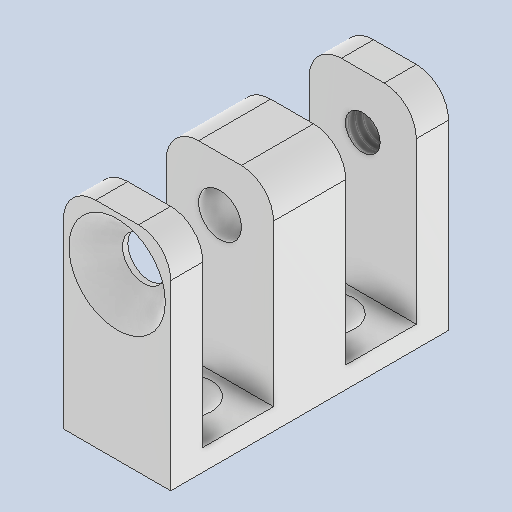
# Autodesk Inventor part: HalterUmlenkrolleDPL
Saved by Autodesk Inventor 2025 (Build 290162010, 162A)
## iProperties
Created: 2024-11-18
Part Number: HalterUmlenkrolleDPL
Material: PC/ABS-Kunststoff, 3DDruck, PLA
Document SubType Name: Modeling
Designer: Admin
Density: 1.1 g/cm^3
Appearance: Glatt - Weiß(2)
Mass: 2.7775 g
Surface Area: 22.2803 cm^2
Volume: 2.525 cm^3
Author: Admin
Autodesk Inventor part; units mm, degrees
ref_plane "YZ Plane" through (0, 0, 0) normal (1, 0, 0) x (0, 1, 0)
ref_plane "XZ Plane" through (0, 0, 0) normal (0, 1, 0) x (-1, 0, 0)
ref_plane "XY Plane" through (0, 0, 0) normal (0, 0, 1) x (1, 0, 0)
sketch "Skizze1" plane through (0, 0, 0) normal (0, 0, 1) x (1, 0, 0)
  line L0 (12.8939, 32.0057) -> (2.8939, 32.0057)
  line L1 (2.8939, 32.0057) -> (2.8939, 29.0057)
  line L2 (2.8939, 29.0057) -> (12.8939, 29.0057)
  line L3 (12.8939, 29.0057) -> (12.8939, 32.0057)
  line L4 (12.8939, 9.0723) -> (2.8939, 9.0723)
  line L5 (2.8939, 9.0723) -> (2.8939, 6.0723)
  line L6 (2.8939, 6.0723) -> (12.8939, 6.0723)
  line L7 (12.8939, 6.0723) -> (12.8939, 9.0723)
  line L8 (2.8939, 15.6723) -> (12.8939, 15.6723)
  line L9 (12.8939, 15.6723) -> (12.8939, 22.4057)
  line L10 (12.8939, 22.4057) -> (2.8939, 22.4057)
  line L11 (2.8939, 22.4057) -> (2.8939, 15.6723)
  line L12 (2.8939, 9.0723) -> (2.8939, 15.6723) construction
  line L13 (2.8939, 22.4057) -> (2.8939, 29.0057) construction
  point P0 (0, 0)
  point P1 (7.8939, 9.0723)
  dimension "d0" = 10
  dimension "d1" = 3
  dimension "d2" = 3
  dimension "d35" = 25.9333
  dimension "d38" = 6.6
  dimension "d39" = 6.7333
  constraints: 28 end point, 7 equal length, 4 collinear, 4 horizontal, 3 perpendicular, 2 vertical, 1 midpoint
  measures "d0" distance of L2.end L1.end
  measures "d1" distance of L0.end L1.end
  measures "d2" distance of L4.end L5.end
  measures "d35" distance between parallel lines of L0 L6
  measures "d38" distance of L8.start L4.end
  measures "d39" distance of L8.end L9.end
extrude "Extrusion1" add sketch "Skizze1" along normal blind 20
fillet "Rundung1" radius 3 6 edges at (12.8939, 7.5723, 20) (12.8939, 30.5057, 20) (2.8939, 30.5057, 20) (2.8939, 7.5723, 20) (12.8939, 19.039, 20) (2.8939, 19.039, 20)
sketch "Skizze2" plane through (2.8939, 6.0723, 0) normal (0, -1, 0) x (1, 0, 0)
  circle A0 centre (5, 15) radius 5 construction
  line L0 (10, 0) -> (10, 17) construction
  line L1 (0, 0) -> (0, 17) construction
  line L2 (3, 20) -> (7, 20) construction
  point P0 (-2.8939, 0)
  constraints: 3 tangent, 1 centre point
hole "Bohrung1" at (7.8939, 6.0723, 15) direction (0, 1, 0) diameter 3.242 end through all countersink diameter 9 countersink angle 90 thread size "M4x0.7" class "6H" standard "ISO Metric profile"
sketch "Skizze3" plane through (2.8939, 29.0057, 0) normal (0, -1, 0) x (1, 0, 0)
  line L0 (0, 0) -> (10, 0) projected
  line L1 (10, 0) -> (10, 2)
  line L2 (10, 0) -> (10, 17) projected
  line L3 (10, 2) -> (0, 2)
  line L4 (0, 0) -> (0, 17) projected
  point P0 (-2.8939, 0)
  dimension "d15" = 2
  constraints: 4 end point, 2 point on line, 1 perpendicular
  measures "d15" distance of L0.end L1.end
extrude "Extrusion2" add sketch "Skizze3" along normal through all
sketch "Skizze4" plane through (2.8939, 29.0057, 2) normal (0, 0, 1) x (1, 0, 0)
  line L0 (5, -16.6333) -> (10, -16.6333) construction
  line L1 (10, -16.6333) -> (10, 0) construction
  line L2 (10, -16.6333) -> (10, -19.9333) construction
  line L3 (5, -3.3) -> (0, -3.3) construction
  line L4 (0, 0) -> (0, -3.3) construction
  line L5 (5, -16.6333) -> (0, -16.6333) construction
  line L6 (0, 0) -> (0, -19.9333) construction
  point P0 (-2.8939, -29.0057)
  dimension "d34" = 13.3333
  constraints: 12 end point, 3 equal length, 3 horizontal, 2 vertical, 1 point on line
  measures "d34" distance of L3.start L0.start
hole "Bohrung2" at (7.8939, 25.7057, 2) at (7.8939, 12.3723, 2) direction (0, 0, -1) diameter 2 end through all countersink diameter 5 countersink angle 90
sketch "Skizze5" plane through (2.8939, 6.0723, 0) normal (0, -1, 0) x (1, 0, 0)
  circle A0 centre (5, 15) radius 4.5 projected
  point P0 (-2.8939, 0)
hole "Bohrung3" at (7.8939, 6.0723, 15) direction (0, 1, 0) diameter 4 depth 22.9333
